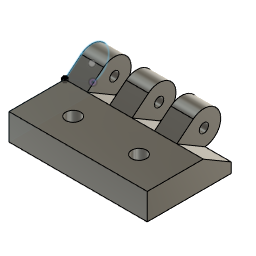
Top Hinge (Autodesk Fusion 360 design; units mm, degrees)
Autodesk Fusion 360 part; units mm, degrees
sketch "Sketch1" plane through (0, 0, 0) normal (0, 0, 1) x (1, 0, 0)
  line L0 (21, 8.5) -> (-21, 8.5)
  line L1 (-21, 8.5) -> (-21, -8.5)
  line L2 (-21, -8.5) -> (21, -8.5)
  line L3 (21, -8.5) -> (21, 8.5)
  line L4 (21, 8.5) -> (-21, -8.5) construction
  line L5 (-21, 8.5) -> (21, -8.5) construction
  dimension "d1" = 17
  dimension "d2" = 42
  constraint horizontal L0
  constraint perpendicular L0 L1
  constraint parallel L0 L2
  constraint parallel L1 L3
  constraint coincident L4 origin
  constraint coincident L5 origin
  measures "d1" distance of L0.start L2.end
  measures "d2" distance of L1.end L2.end
extrude "Extrude1" add sketch "Sketch1" along normal blind 8
sketch "Sketch2" plane through (0, 0, 8) normal (0, 0, 1) x (-1, 0, 0)
  line L0 (-21, 8.5) -> (-21, -8.5)
  line L1 (-21, -8.5) -> (21, -8.5)
  line L2 (21, -8.5) -> (21, 8.5)
  line L3 (21, 8.5) -> (-21, 8.5)
  circle A0 centre (14, 0) radius 3.15
  circle A1 centre (-14, 0) radius 3.15
  dimension "d6" = 6.3
  dimension "d7" = 6.3
  dimension "d8" = 28
  dimension "d9" = 7
  constraint horizontal A0.centre A1.centre
  constraint horizontal origin A1.centre
  measures "d6" diameter of A1
  measures "d7" diameter of A0
  measures "d8" distance of A0.centre A1.centre
  measures "d9" distance of L2 A0.centre
sketch "Sketch3" plane through (21, 0, 0) normal (1, 0, 0) x (0, 1, 0)
  line L0 (-8.5, 0) -> (8.5, 0)
  line L1 (8.5, 0) -> (8.5, 8)
  line L2 (8.5, 8) -> (-8.5, 8)
  line L3 (-8.5, 8) -> (-8.5, 0)
  line L4 (8.5, 8) -> (17, 3)
  line L5 (17, 3) -> (17, 0)
  line L6 (17, 0) -> (8.5, 0)
  dimension "d23" = 8.5
  dimension "d24" = 3
  constraint coincident L1.end L2.start
  constraint perpendicular L2 L5
  constraint coincident L0.end L1.start
  constraint perpendicular L1 L6
  measures "d23" distance of L5.end L0.end
  measures "d24" distance of L4.end L5.end
extrude "Extrude3" add sketch "Sketch3" against normal up to surface (42 mm away) contours L1 L4 L5 L6
sketch "Sketch4" plane through (-21, 0, 0) normal (-1, 0, 0) x (0, -1, 0)
  line L0 (-17, 0) -> (8.5, 0)
  line L1 (8.5, 0) -> (8.5, 8)
  line L2 (8.5, 8) -> (-8.5, 8)
  line L3 (-8.5, 8) -> (-17, 3)
  line L4 (-17, 3) -> (-17, 0)
  line L5 (-8.5, 8) -> (-13.4696, 12.057)
  arc A0 (-13.4696, 12.057) -> (-17, 3) centre (-16.7002, 8.0997) ccw
  constraint coincident L2.end L3.start
  constraint coincident L5.end A0
  constraint coincident L5 A0.start
  constraint tangent L5 A0
extrude "Extrude4" add sketch "Sketch4" against normal blind 6.8 contours L3 L5 A0
extrude "Extrude5" add 1 faces at (-14.2, 12.9899, 7.6857) along direction (1, 0, 0) blind 6.8 from surface at 6.8
extrude "Extrude6" add 1 faces at (-0.6, 12.9899, 7.6857) along direction (1, 0, 0) blind 6.8 from surface at 6.8
sketch "Sketch5" plane through (-21, 0, 0) normal (-1, 0, 0) x (0, -1, 0)
  line L0 (-17, 0) -> (8.5, 0)
  line L1 (8.5, 0) -> (8.5, 8)
  line L2 (8.5, 8) -> (-8.5, 8)
  line L3 (-8.5, 8) -> (-13.4696, 12.057)
  arc A0 (-13.4696, 12.057) -> (-17, 3) centre (-16.7002, 8.0997) ccw
  line L4 (-17, 3) -> (-17, 0)
  circle A1 centre (-16.7002, 8.0997) radius 1.4
  dimension "d35" = 2.8
  constraint concentric A0 A1
  measures "d35" diameter of A1
extrude "Extrude7" cut sketch "Sketch5" against normal up to surface (34 mm away) contours A1
sketch "Sketch8" plane through (0, 0, 8) normal (0, 0, 1) x (-1, 0, 0)
  line L0 (-21, 8.5) -> (-21, -8.5)
  line L1 (-21, -8.5) -> (-13, -8.5)
  line L2 (-13, -8.5) -> (-6.2, -8.5)
  line L3 (-6.2, -8.5) -> (0.6, -8.5)
  line L4 (0.6, -8.5) -> (7.4, -8.5)
  line L5 (7.4, -8.5) -> (14.2, -8.5)
  line L6 (14.2, -8.5) -> (21, -8.5)
  line L7 (21, -8.5) -> (21, 8.5)
  line L8 (21, 8.5) -> (-21, 8.5)
  line L9 (21, 0) -> (-21, 0) construction
  circle A0 centre (10, 0) radius 2.25 construction
  circle A1 centre (-10, 0) radius 2.25 construction
  dimension "d49" = 20
  dimension "d50" = 4.5
  dimension "d51" = 11
  dimension "d52" = 11
  constraint midpoint L0 L9.end
  constraint perpendicular L0 L9
  constraint coincident L9 A0.centre
  constraint coincident L9 A1.centre
  constraint equal A0 A1
  measures "d49" distance of A0.centre A1.centre
  measures "d50" diameter of A0
  measures "d51" distance of L9.start A0.centre
  measures "d52" distance of L9.end A1.centre
hole "Hole3" at (-10, 0, 8) at (10, 0, 8) direction (0, 0, -1) diameter 4.5 depth 10 tip angle 118
